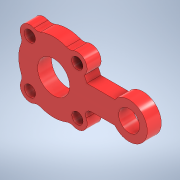
# Autodesk Inventor part: hw13
Saved by Autodesk Inventor 2021 (Build 250183000, 183)
## iProperties
Created: 2022-04-30
Part Number: hw13
Material: Generic
Document SubType Name: Modeling
Designer: authe
Density: 1 g/cm^3
Appearance: Light Red
Author: authe
Autodesk Inventor part; units mm, degrees
ref_plane "YZ Plane" through (0, 0, 0) normal (1, 0, 0) x (0, 1, 0)
ref_plane "XZ Plane" through (0, 0, 0) normal (0, 1, 0) x (-1, 0, 0)
ref_plane "XY Plane" through (0, 0, 0) normal (0, 0, 1) x (1, 0, 0)
sketch "Sketch1" plane through (0, 0, 0) normal (1, 0, 0) x (0, 1, 0)
  point P0 (0, 0)
sketch "Sketch2" plane through (0, 0, 0) normal (0, 0, 1) x (1, 0, 0)
  circle A0 centre (0, 0) radius 11.5
  line L0 (0, 0) -> (16.9235, 17.0175)
  circle A1 centre (16.9235, 17.0175) radius 4
  circle A2 centre (16.9235, 17.0175) radius 7
  circle A3 centre (-17.0175, 16.9235) radius 4
  circle A4 centre (-17.0175, 16.9235) radius 7
  circle A5 centre (-16.9235, -17.0175) radius 4
  circle A6 centre (-16.9235, -17.0175) radius 7
  circle A7 centre (17.0175, -16.9235) radius 4
  circle A8 centre (17.0175, -16.9235) radius 7
  line L1 (0, 0) -> (54, 0)
  circle A9 centre (54, 0) radius 7.5
  circle A10 centre (54, 0) radius 13
  line L2 (34.0355, 0) -> (34.0355, 8)
  line L3 (34.0355, 8) -> (34.0355, -8)
  line L4 (34.0355, -8) -> (43.753, -8)
  line L5 (23.6854, -8) -> (34.0355, -8)
  line L6 (34.0355, 8) -> (43.753, 8)
  line L7 (34.0355, 8) -> (23.6854, 8)
  arc A11 (-19.5919, 13.8621) -> (-21.1769, 11.2933) centre (0, 0) ccw
  arc A12 (11.96, 21.9535) -> (-12.0815, 21.8869) centre (0, 0) ccw
  arc A13 (-21.9535, 11.96) -> (-21.8869, -12.0815) centre (0, 0) ccw
  arc A14 (-11.96, -21.9535) -> (12.0815, -21.8869) centre (0, 0) ccw
  arc A15 (21.9535, -11.96) -> (21.8869, 12.0815) centre (0, 0) ccw
  dimension "d1" = 23
  dimension "d4" = 8
  dimension "d5" = 14
  dimension "d8" = 360
  dimension "d10" = 54
  dimension "d11" = 15
  dimension "d12" = 26
  dimension "d13" = 8
  dimension "d14" = 16
  constraints: 23 point on circle, 16 end point, 15 centre point, 10 coincident, 3 horizontal, 3 point on line, 2 perpendicular, 1 collinear, 20 other
  measures "d1" diameter of A0
  measures "d4" diameter of A1
  measures "d5" diameter of A2
  measures "d10" distance of L0.start L1.end
  measures "d11" diameter of A9
  measures "d12" diameter of A10
  measures "d13" distance of L2.start L2.end
  measures "d14" distance of L2.end L3.end
extrude "Extrusion1" add sketch "Sketch2" along normal blind 10 contours L1 A15 A8 A14 A6 A13 A4 A12 A2 L0 A0 | A0 L0 A2 A15 L1 | A15 L7 L2 L1 | L1 L3 L5 A15 | A2 | L2 L6 A10 L1 | L1 A10 L4 L3 | A10 | A8 | A4 | A6 | A9
extrude "Extrusion2" cut sketch "Sketch2" along normal blind 10 contours A9
fillet "Fillet1" radius 4 2 edges at (23.6854, -8, 5) (21.9535, -11.96, 5)
fillet "Fillet2" radius 6 6 edges at (11.96, 21.9535, 5) (-12.0815, 21.8869, 5) (-21.9535, 11.96, 5) (-21.8869, -12.0815, 5) (-11.96, -21.9535, 5) (12.0815, -21.8869, 5)
body "Solid1"
